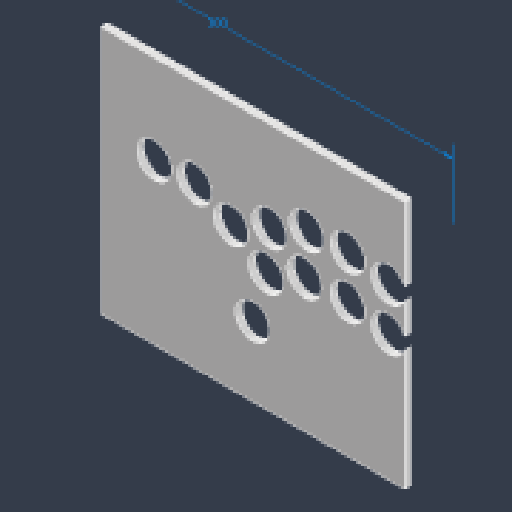
# Autodesk Inventor part: Top Plate Sanwa
Saved by Autodesk Inventor 2023.4 (Build 274418000, 418)
## iProperties
Created: 2024-02-20
Part Number: Top Plate Sanwa
Material: Generic
Document SubType Name: Modeling
Designer: JoaoSilva
Density: 1 g/cm^3
Appearance: Default
Author: JoaoSilva
Autodesk Inventor part; units mm, degrees
ref_plane "YZ Plane" through (0, 0, 0) normal (1, 0, 0) x (0, 1, 0)
ref_plane "XZ Plane" through (0, 0, 0) normal (0, 1, 0) x (-1, 0, 0)
ref_plane "XY Plane" through (0, 0, 0) normal (0, 0, 1) x (1, 0, 0)
sketch "Sketch1" plane through (0, 0, 0) normal (0, 0, 1) x (1, 0, 0)
  line L0 (-150, 90) -> (150, 90)
  line L1 (150, 90) -> (150, -90)
  line L2 (150, -90) -> (-150, -90)
  line L3 (-150, -90) -> (-150, 90)
  line L4 (-150, 90) -> (150, -90) construction
  line L5 (150, 90) -> (-150, -90) construction
  point P0 (0, 0)
  dimension "d0" = 300
  dimension "d1" = 180
  constraints: 12 end point, 2 midpoint, 2 parallel, 1 horizontal, 1 perpendicular
  measures "d0" distance of L0.start L0.end
  measures "d1" distance of L2.end L0.start
extrude "Extrusion1" add sketch "Sketch1" along normal blind 5
sketch "Sketch2" plane through (0, 0, 5) normal (0, 0, 1) x (1, 0, 0)
  line L0 (-150, -90) -> (150, -90) projected
  point P0 (0, 0)
  point P1 (0, -39.6)
  point P2 (-15.5, 12.8)
  point P3 (-41.8, 25.7)
  point P4 (-71.3, 25.6)
  point P5 (9.7, -4.6)
  point P6 (12.3, 24.8)
  point P7 (37.5, 6.4)
  point P8 (39.2, 36.5)
  point P9 (68.8, 6.7)
  point P10 (68.8, 37.7)
  point P11 (98.3, 1.7)
  point P12 (98.3, 32.7)
  dimension "d4" = 50.4
  dimension "d5" = 15.5
  dimension "d6" = 26.3
  dimension "d7" = 29.5
  dimension "d11" = 52.4
  dimension "d12" = 65.3
  dimension "d13" = 65.2
  dimension "d14" = 9.7
  dimension "d15" = 29.4
  dimension "d16" = 2.6
  dimension "d17" = 26.9
  dimension "d18" = 29.6
  dimension "d19" = 29.5
  dimension "d20" = 1.7
  dimension "d22" = 46
  dimension "d23" = 30.1
  dimension "d24" = 96.7
  dimension "d25" = 91.7
  dimension "d26" = 31
  dimension "d27" = 31
  dimension "d28" = 35
  constraints: 3 vertical alignment
  measures "d4" distance from line of L0 point (0, -39.6)
  measures "d5" horizontal distance of point (0, -39.6) point (-15.5, 12.8)
  measures "d6" horizontal distance of point (-41.8, 25.7) point (-15.5, 12.8)
  measures "d7" horizontal distance of point (-71.3, 25.6) point (-41.8, 25.7)
  measures "d11" vertical distance of point (0, -39.6) point (-15.5, 12.8)
  measures "d12" vertical distance of point (0, -39.6) point (-41.8, 25.7)
  measures "d13" vertical distance of point (-71.3, 25.6) point (0, -39.6)
  measures "d14" horizontal distance of point (9.7, -4.6) point (0, -39.6)
  measures "d15" vertical distance of point (12.3, 24.8) point (9.7, -4.6)
  measures "d16" horizontal distance of point (12.3, 24.8) point (9.7, -4.6)
  measures "d17" horizontal distance of point (39.2, 36.5) point (12.3, 24.8)
  measures "d18" horizontal distance of point (68.8, 37.7) point (39.2, 36.5)
  measures "d19" horizontal distance of point (98.3, 32.7) point (68.8, 37.7)
  measures "d20" horizontal distance of point (39.2, 36.5) point (37.5, 6.4)
  measures "d22" vertical distance of point (37.5, 6.4) point (0, -39.6)
  measures "d23" vertical distance of point (39.2, 36.5) point (37.5, 6.4)
  measures "d24" distance from line of L0 point (68.8, 6.7)
  measures "d25" distance from line of L0 point (98.3, 1.7)
  measures "d26" distance of point (98.3, 32.7) point (98.3, 1.7)
  measures "d27" distance of point (68.8, 6.7) point (68.8, 37.7)
  measures "d28" vertical distance of point (9.7, -4.6) point (0, -39.6)
hole "Hole1" at (0, -39.6, 5) at (-15.5, 12.8, 5) at (-41.8, 25.7, 5) at (-71.3, 25.6, 5) at (9.7, -4.6, 5) at (12.3, 24.8, 5) at (37.5, 6.4, 5) at (39.2, 36.5, 5) at (68.8, 6.7, 5) at (68.8, 37.7, 5) at (98.3, 1.7, 5) at (98.3, 32.7, 5) direction (0, 0, -1) diameter 25 end through all clearance for "Socket Head Cap Screw ISO 4762" size "M24" standard "ISO"
sketch "Sketch5" plane through (0, 0, 5) normal (0, 0, 1) x (1, 0, 0)
  circle A0 centre (0, -39.6) radius 12.5 projected
  point P0 (0, 0)
hole "Hole2" at (0, -39.6, 5) direction (0, 0, -1) diameter 31 end through all clearance for "Socket Head Cap Screw ISO 4762" size "M30" standard "ISO"
body "Solid1"
